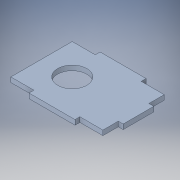
# Autodesk Inventor part: HOMBRO_SOST.COJ
Saved by Autodesk Inventor 2019 (Build 230136000, 136)
## iProperties
Created: 2020-02-12
Part Number: HOMBRO_SOST.COJ
Material: Genérico
Document SubType Name: Modeling
Designer: omar-
Density: 1 g/cm^3
Appearance: Valor por defecto
Author: omar-
Autodesk Inventor part; units mm, degrees
ref_plane "YZ Plane" through (0, 0, 0) normal (1, 0, 0) x (0, 1, 0)
ref_plane "XZ Plane" through (0, 0, 0) normal (0, 1, 0) x (-1, 0, 0)
ref_plane "XY Plane" through (0, 0, 0) normal (0, 0, 1) x (1, 0, 0)
sketch "Boceto1" plane through (0, 0, 0) normal (0, 1, 0) x (-1, 0, 0)
  circle A0 centre (0, 0) radius 9.5
  line L0 (20, 20) -> (-40, 20)
  line L1 (-40, 20) -> (-40, -20)
  line L2 (-40, -20) -> (20, -20)
  line L3 (20, -20) -> (20, 20)
  line L4 (5, 23.18) -> (-25, 23.18)
  line L5 (-25, 23.18) -> (-25, 20)
  line L6 (-25, 20) -> (5, 20)
  line L7 (5, 20) -> (5, 23.18)
  line L8 (5, -20) -> (-25, -20)
  line L9 (-25, -20) -> (-25, -23.18)
  line L10 (-25, -23.18) -> (5, -23.18)
  line L11 (5, -23.18) -> (5, -20)
  line L12 (-40, 10) -> (-43.18, 10)
  line L13 (-43.18, 10) -> (-43.18, -10)
  line L14 (-43.18, -10) -> (-40, -10)
  line L15 (-40, -10) -> (-40, 10)
  dimension "d0" = 19
  dimension "d17" = 40
  dimension "d18" = 60
  dimension "d19" = 20
  dimension "d20" = 20
  dimension "d21" = 3.18
  dimension "d22" = 30
  dimension "d23" = 15
  dimension "d24" = 20
  dimension "d25" = 10
  dimension "d26" = 3.18
  constraints: 32 end point, 8 parallel, 4 coincident, 4 collinear, 4 horizontal, 4 perpendicular, 2 equal length, 1 centre point
  measures "d0" diameter of A0
  measures "d17" distance of L2.end L0.start
  measures "d18" distance of L1.end L2.end
  measures "d19" distance from line of L2 point (0, 0)
  measures "d20" distance from line of L3 point (0, 0)
  measures "d21" distance of L10.end L8.start
  measures "d22" distance of L9.end L10.end
  measures "d23" distance between parallel lines of L11 L3
  measures "d24" distance of L12.end L13.end
  measures "d25" distance between parallel lines of L12 L0
  measures "d26" distance of L13.end L14.end
extrude "Extrusión1" add sketch "Boceto1" along normal blind 3.18
